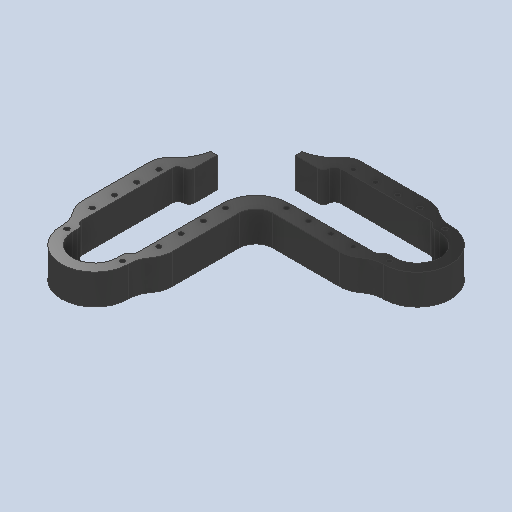
# Autodesk Inventor part: Gearbox Cover Large
Saved by Autodesk Inventor 2025.1 (Build 291241020, 241B)
## iProperties
Created: 2023-09-21
Part Number: Gearbox Cover Large
Material: Generic
Document SubType Name: Modeling
Designer: lando
Density: 1 g/cm^3
Appearance: Default
Author: lando
Autodesk Inventor part; units mm, degrees
ref_plane "YZ Plane" through (0, 0, 0) normal (1, 0, 0) x (0, 1, 0)
ref_plane "XZ Plane" through (0, 0, 0) normal (0, 1, 0) x (-1, 0, 0)
ref_plane "XY Plane" through (0, 0, 0) normal (0, 0, 1) x (1, 0, 0)
ref_plane "Work Plane1" through (153.3626, 3.175, 315.1376) normal (0, 1, 0) x (1, 0, 0)
sketch "Sketch2" plane through (153.3626, 3.175, 315.1376) normal (0, 1, 0) x (1, 0, 0)
  line L0 (-69.85, 187.175) -> (-77.0435, 187.175)
  circle A0 centre (-88.9, 139.7) radius 2.65
  circle A1 centre (-88.9, 114.3) radius 2.65
  line L1 (-101.6, 142.5126) -> (-101.6, 66.6752)
  line L2 (-76.2, 34.5627) -> (-76.2, 28.5752)
  line L3 (-57.0148, 33.9239) -> (-71.3794, 33.9239) construction
  arc A2 (-82.55, 45.5613) -> (-79.375, 40.062) centre (-76.2, 45.5613) ccw
  line L4 (-76.2, 155.2126) -> (-76.2, 155.2126)
  line L5 (-19.05, 45.5613) -> (-19.05, 142.5127)
  line L6 (-25.4, 34.5627) -> (-25.4, 28.5752)
  arc A3 (-22.225, 40.062) -> (-25.4, 34.5627) centre (-19.05, 34.5627) ccw
  arc A4 (-22.225, 40.062) -> (-19.05, 45.5613) centre (-25.4, 45.5613) ccw
  arc A5 (19.0506, 161.5633) -> (0, 142.5127) centre (19.0506, 142.5127) ccw
  arc A6 (19.0506, 180.6133) -> (-19.05, 142.5127) centre (19.0506, 142.5127) ccw
  line L7 (-24.798, 231.625) -> (-24.798, 238.8185)
  circle A7 centre (22.0226, 250.7457) radius 2.65
  circle A8 centre (47.4226, 250.7457) radius 2.65
  arc A9 (133.2003, 174.2609) -> (132.8314, 250.6758) centre (133.2003, 212.4693) ccw
  line L8 (116.2139, 244.3252) -> (13.5144, 244.3252)
  arc A10 (133.2003, 186.9633) -> (133.2003, 237.9752) centre (133.2003, 212.4693) ccw
  line L9 (127.2124, 237.9752) -> (133.2003, 237.9752)
  arc A11 (121.7132, 241.1502) -> (127.2124, 237.9752) centre (127.2124, 244.3252) ccw
  arc A12 (121.7132, 241.1502) -> (116.2139, 244.3252) centre (116.2139, 237.9752) ccw
  line L10 (0.8144, 231.625) -> (-24.798, 231.625)
  line L11 (116.2145, 180.6133) -> (19.0506, 180.6133)
  arc A13 (127.213, 186.9633) -> (121.7138, 183.7883) centre (127.213, 180.6133) ccw
  arc A14 (116.2145, 180.6133) -> (121.7138, 183.7883) centre (116.2145, 186.9633) ccw
  line L12 (127.213, 186.9633) -> (133.2003, 186.9633)
  arc A15 (-24.798, 238.8185) -> (4.1198, 256.1306) centre (-34.9551, 288.5928) ccw
  arc A16 (18.7729, 263.0074) -> (4.1198, 256.1306) centre (18.7729, 243.9574) ccw
  line L13 (0, 142.5127) -> (0, 66.6752)
  arc A17 (-94.6727, 157.2075) -> (-101.6, 142.5126) centre (-82.55, 142.5126) ccw
  arc A18 (-94.6727, 157.2075) -> (-77.0435, 187.175) centre (-127, 196.3941) ccw
  line L14 (19.0506, 161.5633) -> (95.1006, 161.5633)
  line L15 (-101.6, 66.6752) -> (-101.6, 47.6252) construction
  line L16 (-101.6, 47.6252) -> (-88.9, 47.6252) construction
  line L17 (-88.9, 47.6252) -> (-88.9, 28.5752) construction
  spline S0 degree 3 poles (-101.6, 66.6752) (-101.6, 47.6252) (-88.9, 47.6252) (-88.9, 28.5752) knots 1 1 1 1 2 2 2 2
  spline S1 degree 3 poles (0, 66.6752) (0, 47.6252) (-12.7, 47.6252) (-12.7, 28.5752) knots 1 1 1 1 2 2 2 2
  line L18 (0, 66.6752) -> (0, 47.6252) construction
  line L19 (0, 47.6252) -> (-12.7, 47.6252) construction
  line L20 (-12.7, 47.6252) -> (-12.7, 28.5752) construction
  spline S2 degree 3 poles (94.6105, 263.0074) (113.6596, 263.1913) (113.7823, 250.4919) (132.8314, 250.6758) knots 1 1 1 1 2 2 2 2
  line L21 (94.6105, 263.0074) -> (113.6596, 263.1913) construction
  line L22 (113.6596, 263.1913) -> (113.7823, 250.4919) construction
  line L23 (113.7823, 250.4919) -> (132.8314, 250.6758) construction
  spline S3 degree 3 poles (95.1006, 161.5633) (114.1506, 161.5633) (114.1506, 174.2609) (133.2003, 174.2609) knots 1 1 1 1 2 2 2 2
  line L24 (95.1006, 161.5633) -> (114.1506, 161.5633) construction
  line L25 (114.1506, 161.5633) -> (114.1506, 174.2609) construction
  line L26 (114.1506, 174.2609) -> (133.2003, 174.2609) construction
  circle A19 centre (-88.9, 88.9) radius 2.65
  circle A20 centre (-88.9, 63.5) radius 2.65
  circle A21 centre (-82.55, 28.5752) radius 2.65
  circle A22 centre (-19.05, 28.5752) radius 2.65
  circle A23 centre (-12.7, 63.5) radius 2.65
  circle A24 centre (-12.7, 88.9) radius 2.65
  circle A25 centre (-12.7, 114.3) radius 2.65
  circle A26 centre (-12.7, 139.7) radius 2.65
  circle A27 centre (22.075, 174.475) radius 2.65
  circle A28 centre (47.475, 174.475) radius 2.65
  circle A29 centre (72.875, 174.475) radius 2.65
  circle A30 centre (98.275, 174.475) radius 2.65
  circle A31 centre (133.2, 180.825) radius 2.65
  circle A32 centre (133.2, 244.325) radius 2.65
  circle A33 centre (98.2226, 250.7457) radius 2.65
  circle A34 centre (72.8226, 250.7457) radius 2.65
  arc A35 (-88.9, 28.5752) -> (-12.7, 28.5752) centre (-50.8, 28.5752) ccw
  line L27 (94.6105, 263.0074) -> (18.7729, 263.0074)
  line L28 (-69.85, 187.175) -> (-69.85, 161.5626)
  line L29 (-82.55, 148.8626) -> (-82.55, 45.5613)
  arc A36 (-76.2, 34.5627) -> (-79.375, 40.062) centre (-82.55, 34.5627) ccw
  arc A37 (0.8144, 231.625) -> (7.1644, 237.9751) centre (0.8144, 237.975) ccw
  arc A38 (13.5144, 244.3252) -> (7.1644, 237.9751) centre (13.5144, 237.9752) ccw
  arc A39 (-76.2, 155.2126) -> (-69.85, 161.5626) centre (-76.2, 161.5626) ccw
  arc A40 (-76.2, 155.2126) -> (-82.55, 148.8626) centre (-76.2, 148.8626) ccw
  arc A41 (-76.2, 28.5752) -> (-25.4, 28.5752) centre (-50.8, 28.5752) ccw
  point P0 (19.2624, 180.825)
  point P1 (-19.05, 142.5126)
  point P2 (-153.3626, 315.1376)
  dimension "d62" = 5.3
  dimension "d64" = 7.1935
  dimension "d65" = 25.6124
  dimension "d72" = 12.7
  dimension "d73" = 19.05
  dimension "d74" = 19.05
  dimension "d75" = 6.4205
  dimension "d76" = 25.4
  dimension "d77" = 25.4
  dimension "d78" = 25.4
  dimension "d104" = 6.35
  dimension "d105" = 6.35
  dimension "d106" = 6.35
  dimension "d107" = 6.35
  dimension "d109" = 6.35
  dimension "d110" = 6.35
  dimension "d111" = 19.05
  dimension "d112" = 19.05
  dimension "d114" = 34.9248
  dimension "d115" = 31.75
  dimension "d116" = 25.4
  dimension "d117" = 25.4
  dimension "d118" = 25.4
  dimension "d122" = 38.1
  dimension "d124" = 5.3
  dimension "d125" = 6.35
  dimension "d126" = 6.35
  dimension "d127" = 6.35
  dimension "d128" = 5.9875
  dimension "d129" = 12.7
  dimension "d130" = 19.05
  dimension "d131" = 19.05
  dimension "d132" = 16.9861
  dimension "d133" = 6.35
  dimension "d134" = 96.9515
  dimension "d135" = 5.4993
  dimension "d136" = 25.4
  dimension "d137" = 102.5626
  dimension "d138" = 286.5624
  dimension "d139" = 25.4
  dimension "d140" = 5.9875
  dimension "d141" = 12.7
  dimension "d142" = 12.7
  dimension "d143" = 19.05
  dimension "d144" = 19.05
  dimension "d145" = 12.7
  dimension "d146" = 25.4
  dimension "d147" = 19.0506
  dimension "d148" = 25.4
  dimension "d149" = 25.4
  dimension "d150" = 25.4
  dimension "d151" = 5.3
  dimension "d152" = 19.05
  dimension "d153" = 12.6976
  dimension "d154" = 19.0497
  dimension "d155" = 38.2083
  dimension "d156" = 25.5059
  dimension "d157" = 6.35
  dimension "d158" = 6.35
  dimension "d159" = 97.1639
  dimension "d160" = 10.9985
  dimension "d161" = 5.4993
  dimension "d162" = 5.9873
  dimension "d163" = 5.3
  constraints: 46 point on circle, 42 centre point, 36 end point, 22 tangent, 16 equal radius, 9 horizontal, 7 horizontal alignment, 7 perpendicular, 7 vertical, 5 vertical alignment, 1 point on line, 20 other
  measures "d62" diameter of A0
  measures "d64" distance of L7.start L7.end
  measures "d65" distance of L10.start L7.start
  measures "d72" distance of L21.end L22.end
  measures "d73" distance of L21.start L21.end
  measures "d74" distance of L22.end L23.end
  measures "d75" distance from line of L8 A7.centre
  measures "d76" distance of A8.centre A7.centre
  measures "d77" distance of A34.centre A8.centre
  measures "d78" distance of A33.centre A34.centre
  measures "d104" radius of A2
  measures "d105" radius of A36
  measures "d106" radius of A38
  measures "d107" radius of A37
  measures "d109" radius of A39
  measures "d110" radius of A40
  measures "d111" distance between parallel lines of L29 L1
  measures "d112" distance between parallel lines of L5 L13
  measures "d114" vertical distance of A22.centre A23.centre
  measures "d115" distance of A35.centre A22.centre
  measures "d116" distance of A19.centre A20.centre
  measures "d117" distance of A1.centre A19.centre
  measures "d118" distance of A0.centre A1.centre
  measures "d122" radius of A35
  measures "d124" diameter of A22
  measures "d125" distance from line of L5 A23.centre
  measures "d126" radius of A3
  measures "d127" radius of A4
  measures "d128" distance of L6.start L6.end
  measures "d129" distance of L18.end L19.end
  measures "d130" distance of L19.end L20.end
  measures "d131" distance of L13.end L18.end
  measures "d132" vertical distance of L6.end L5.start
  measures "d133" horizontal distance of L5.start L6.start
  measures "d134" distance of L5.start L5.end
  measures "d135" vertical distance of A3.start L6.start
  measures "d136" distance of A23.centre A24.centre
  measures "d137" horizontal distance of A35.centre point (-153.363, 315.138)
  measures "d138" vertical distance of point (-153.363, 315.138) A35.centre
  measures "d139" radius of A41
  measures "d140" distance of L2.start L2.end
  measures "d141" distance of L20.end L6.end
  measures "d142" distance of L2.end L17.end
  measures "d143" distance of L16.end L17.end
  measures "d144" distance of L1.end L15.end
  measures "d145" distance of L15.end L16.end
  measures "d146" distance of A25.centre A24.centre
  measures "d147" radius of A5
  measures "d148" distance of A28.centre A27.centre
  measures "d149" distance of A29.centre A28.centre
  measures "d150" distance of A30.centre A29.centre
  measures "d151" diameter of A27
  measures "d152" distance of L14.end L24.end
  measures "d153" distance of L24.end L25.end
  measures "d154" distance of L25.end L26.end
  measures "d155" radius of A9
  measures "d156" radius of A10
  measures "d157" radius of A14
  measures "d158" radius of A13
  measures "d159" distance of L11.start L11.end
  measures "d160" horizontal distance of L11.start L12.start
  measures "d161" horizontal distance of L12.start A13.end
  measures "d162" distance of L12.start L12.end
  measures "d163" diameter of A31
extrude "Extrusion2" add sketch "Sketch2" along normal blind 34.417
body "Solid1"
